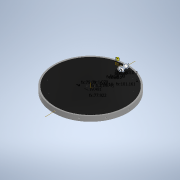
# Autodesk Inventor part: RotorBody
Saved by Autodesk Inventor 2022.2 (Build 262287000, 287)
## iProperties
Created: 2022-07-28
Part Number: RotorBody
Material: ABS Plastic
Document SubType Name: Modeling
Designer: ABL
Density: 1.06 g/cm^3
Appearance: Smooth - Black
Author: ABL
Autodesk Inventor part; units mm, degrees
ref_plane "YZ Plane" through (0, 0, 0) normal (1, 0, 0) x (0, 1, 0)
ref_plane "XZ Plane" through (0, 0, 0) normal (0, 1, 0) x (-1, 0, 0)
ref_plane "XY Plane" through (0, 0, 0) normal (0, 0, 1) x (1, 0, 0)
sketch "Sketch2" plane through (0, 0, 0) normal (0, 1, 0) x (-1, 0, 0)
  circle A0 centre (0, 0) radius 101.16113
  circle A1 centre (0, 0) radius 4.2
  dimension "d4" = 202.32226
  dimension "d101" = 8.4
  constraints: 2 centre point, 2 coincident
  measures "d4" diameter of A0
  measures "d101" diameter of A1
extrude "Extrusion1" add sketch "Sketch2" along normal blind 14.1
ref_plane "Work Plane4" through (-26.182427, 0, -97.714148) normal (-0.258819, 0, -0.9659258) x (0, -1, 0)
sketch "Sketch13" plane through (-27.256526, 0, -101.72274) normal (-0.258819, 0, -0.9659258) x (0, -1, 0)
  line L0 (-14.1, 101.16113) -> (-14.1, -101.16113) construction
  line L1 (0, 0) -> (-14.1, 0) construction
  line L2 (0, 0.05) -> (-14.1, 0.05)
  line L3 (-14.1, 0.05) -> (-14.1, -0.05)
  line L4 (-14.1, -0.05) -> (0, -0.05)
  line L5 (0, -0.05) -> (0, 0.05)
  line L6 (0, 0.05) -> (-14.1, -0.05) construction
  line L7 (-14.1, 0.05) -> (0, -0.05) construction
  point P0 (-7.05, 0)
  dimension "d136" = 0.1
  dimension "d139" = 7.05
  dimension "d140" = 2.05
  dimension "d141" = 4.2
  dimension "d142" = 3.8
  dimension "d146" = 4.1
  dimension "d147" = 4.3
  dimension "d153" = 4.2
  constraints: 8 end point, 2 parallel, 1 horizontal, 1 perpendicular
  measures "d153" distance of L2.end L3.end
sketch "Sketch10" plane through (0, 0, 0) normal (0, -1, 0) x (1, 0, 0)
  line L0 (0, 0) -> (-27.256526, -101.72274)
  line L1 (0, 0) -> (105.31113, 0) construction
  arc A0 (-27.256526, -101.72274) -> (30.042126, -100.935151) centre (0, 0) ccw
  line L2 (0, 0) -> (30.042126, -100.935151)
  line L3 (0, 0) -> (-27.256526, -101.72274) construction
  dimension "d96" = 105.31113
  dimension "d97" = 105
  dimension "d98" = 31.575
  constraints: 8 end point, 2 point on circle, 1 centre point, 1 coincident, 1 equal length, 1 horizontal
  measures "d96" distance of L0.start L0.end
  measures "d97" angle of L0 L1
  measures "d98" angle of L3 L2
sketch "Sketch8" plane through (0, 0, 0) normal (0, 1, 0) x (-1, 0, 0)
  circle A0 centre (0, 0) radius 105.31113
  circle A1 centre (0, 0) radius 101.21113
  dimension "d81" = 210.62226
  dimension "d82" = 202.42226
  constraints: 2 centre point, 2 coincident
  measures "d81" diameter of A0
  measures "d82" diameter of A1
extrude "Extrusion2" add sketch "Sketch8" along normal blind 14.1 separate body
sketch "Sketch1" plane through (0, 0, 0) normal (0, 1, 0) x (-1, 0, 0)
  circle A0 centre (0, 0) radius 38.96113 construction
  arc A1 (-26.182427, -97.714148) -> (26.182427, -97.714148) centre (0, 0) ccw
  line L0 (0, 0) -> (26.182427, -97.714148)
  line L1 (0, 0) -> (101.16113, 0) construction
  line L2 (0, 0) -> (-26.182427, -97.714148)
  line L3 (26.182427, -97.714148) -> (10.083882, -37.633562)
  line L4 (-26.182427, -97.714148) -> (-10.083882, -37.633562)
  line L5 (-9.168017, -38.203527) -> (0.974298, -39.286784)
  line L6 (0.974298, -39.286784) -> (-5.419042, -99.14633)
  line L7 (-5.419042, -99.14633) -> (-15.561357, -98.063073)
  line L8 (-15.561357, -98.063073) -> (-9.168017, -38.203527)
  line L9 (0, 0) -> (0, -101.16113) construction
  line L10 (9.075232, -38.016047) -> (2.9495, -38.972812)
  line L11 (2.9495, -38.972812) -> (12.239385, -98.4517)
  line L12 (12.239385, -98.4517) -> (18.365118, -97.494934)
  line L13 (18.365118, -97.494934) -> (9.075232, -38.016047)
  line L14 (-4.098764, -38.744933) -> (0, 0) construction
  circle A2 centre (-2.049382, -19.372466) radius 2.6
  circle A3 centre (0, 0) radius 101.16113 construction
  line L15 (5.352348, -87.575309) -> (0.955193, -87.733517)
  line L16 (0.955193, -87.733517) -> (1.012724, -89.332482)
  line L17 (1.012724, -89.332482) -> (5.409878, -89.174274)
  line L18 (5.409878, -89.174274) -> (5.352348, -87.575309)
  line L19 (0, 0) -> (3.153771, -87.654413) construction
  line L20 (0.955193, -87.733517) -> (-4.141944, -87.189113) construction
  line L21 (5.352348, -87.575309) -> (10.417072, -86.78426) construction
  line L22 (3.211301, -89.253378) -> (3.637384, -101.095715) construction
  line L23 (-4.098764, -38.744933) -> (-5.150777, -48.689442) construction
  line L24 (5.381113, -88.374792) -> (0.983959, -88.532999) construction
  point P0 (6.012366, -38.49443)
  point P1 (3.182536, -88.453895)
  dimension "d0" = 77.92226
  dimension "d1" = 101.16113
  dimension "d2" = 75
  dimension "d3" = 30
  dimension "d7" = 10.2
  dimension "d8" = 60.2
  dimension "d9" = 6.2
  dimension "d10" = 60.2
  dimension "d11" = 2
  dimension "d15" = 1.07874
  dimension "d16" = 1.07874
  dimension "d17" = 5.2
  dimension "d66" = 4.4
  dimension "d67" = 1.6
  dimension "d79" = 90
  dimension "d80" = 11.85
  dimension "d108" = 19.48057
  dimension "d122" = 10
  constraints: 50 end point, 7 midpoint, 7 perpendicular, 7 point on circle, 4 parallel, 4 point on line, 3 centre point, 3 coincident, 2 collinear, 2 equal length, 2 tangent, 1 horizontal
  measures "d0" diameter of A0
  measures "d1" radius of A1
  measures "d2" angle of L0 L1
  measures "d3" angle of L2 L0
  measures "d7" distance of L6.end L7.end
  measures "d8" distance of L5.end L6.end
  measures "d9" distance of L12.end L11.end
  measures "d10" distance of L11.end L10.end
  measures "d11" distance of L10.end L5.end
  measures "d15" distance of L5.start L4.end
  measures "d16" distance of L3.end L10.start
  measures "d17" diameter of A2
  measures "d66" distance of L15.start L15.end
  measures "d67" distance of L15.end L16.end
  measures "d79" angle of L19 L15
  measures "d80" distance of L22.start L22.end
  measures "d108" distance of A0.centre A2.centre
  measures "d122" distance of L14.start L23.end
extrude "driveMagnet_slot" cut sketch "Sketch1" along normal blind 10.1 contours L5 L6 L7 L8 bodies 1
extrude "halbachMagnet_slot" cut sketch "Sketch1" along normal blind 12.1 contours L13 L12 L11 L10 bodies 1
sketch "Sketch4" plane through (-12.239385, 0, -98.4517) normal (0.154317, 0, 0.9880214) x (0.9880214, 0, -0.154317)
  line L0 (0, 0) -> (0, 12.1) projected
  line L1 (0, 2) -> (-6.2, 2)
  line L2 (-6.2, 2) -> (-6.2, 12.2)
  line L3 (-6.2, 12.2) -> (0, 12.2)
  line L4 (0, 12.2) -> (0, 2)
  line L5 (0, 0) -> (-6.2, 0) projected
  point P0 (-3.1, 0)
  point P1 (0, 12.1)
  dimension "d31" = 6.2
  dimension "halbachMagnet_slotHeight" = 10.2
  dimension "d33" = 2
  constraints: 8 end point, 2 parallel, 1 horizontal, 1 perpendicular, 1 point on line
  measures "d31" distance of L2.end L3.end
  measures "halbachMagnet_slotHeight" distance of L1.end L2.end
  measures "d33" distance between parallel lines of L5 L1
extrude "halbachMagnet_opening" cut sketch "Sketch4" against normal through all bodies 1
extrude "halbachMagnet_roof" add sketch "Sketch1" along normal blind 2 contours L13 L12 L11 L10 bodies 1
extrude "halbachMagnet_slotTopSurfaceIndent" cut sketch "Sketch1" along normal blind 0.2 contours L13 L12 L11 L10 bodies 1
extrude "sensorMagnet_slot" cut sketch "Sketch1" along normal blind 2.766667 contours A2 bodies 1
extrude "rotorBandNut_slot" cut sketch "Sketch1" against normal blind 9.2 from surface at 14.1 contours L18 L17 L16 L15 bodies 1
hole "rotorBandNut_removalHole" at (-3.182536, 0, -88.453895) direction (0, 1, 0) diameter 1.4 depth 4.9 bodies 1
pattern_circular "Sketch1_Pattern" count 12 over 360 about axis through (0, -10, 0) along (0, 1, 0) of "rotorBandNut_removalHole", "rotorBandNut_slot", "sensorMagnet_slot", "halbachMagnet_roof", "halbachMagnet_opening", "halbachMagnet_slot", "driveMagnet_slot", "halbachMagnet_slotTopSurfaceIndent" bodies 1
sketch "Sketch7" plane through (-5.352348, 0, -87.575309) normal (-0.0359563, 0, -0.9993534) x (-0.9993534, 0, 0.0359563)
  line L0 (-2.2, 4.9) -> (-2.2, 7) construction
  line L1 (-4.4, 4.9) -> (0, 4.9) projected
  point P0 (-2.2, 0)
  dimension "d71" = 2.1
  constraints: 2 end point, 1 coincident, 1 midpoint, 1 vertical
  measures "d71" distance of L0.start L0.end
ref_plane "Work Plane2" through (-3.786602, 0, -105.243032) normal (0.0359563, 0, 0.9993534) x (0, 1, 0)
ref_plane "Work Plane1" through (-5.352348, 9.5, -87.575309) normal (0.0359563, 0, 0.9993534) x (0, 1, 0)
sketch "Sketch9" plane through (-3.786602, 0, -105.243032) normal (0.0359563, 0, 0.9993534) x (0, 1, 0)
  line L0 (0, 0) -> (7.05, 0) construction
  dimension "d85" = 7.05
  constraints: 2 coincident, 2 end point, 1 horizontal
  measures "d85" distance of L0.start L0.end
hole "rotorBandBolt_hole" at (-3.786602, 7.05, -105.243032) direction (0.0359563, 0, 0.9993534) diameter 2.4 depth 24 counterbore diameter 4.08 counterbore depth 2.1 bodies 2 1
sketch "Sketch18" plane through (-0.955193, 4.9, -87.733517) normal (-0.0359563, 0, -0.9993534) x (-0.9993534, 0, 0.0359563)
  line L0 (0, 0.879829) -> (0, 3.420171)
  line L1 (0, 3.420171) -> (2.2, 4.690341)
  line L2 (2.2, 4.690341) -> (4.4, 3.420171)
  line L3 (4.4, 3.420171) -> (4.4, 0.879829)
  line L4 (4.4, 0.879829) -> (2.2, -0.390341)
  line L5 (2.2, -0.390341) -> (0, 0.879829)
  circle A0 centre (2.2, 2.15) radius 1.2
  line L6 (0, 9.2) -> (4.4, 9.2)
  line L7 (0, 9.2) -> (0, 0)
  line L8 (0, 0) -> (4.4, 0)
  line L9 (4.4, 0) -> (4.4, 9.2)
  point P0 (2.2, -4.9)
  dimension "d176" = 4.4
  constraints: 12 end point, 1 coincident, 1 vertical, 13 other
  measures "d176" distance between parallel lines of L3 L0
extrude "rotorBandNut_hexCutaway" cut sketch "Sketch18" along normal up to surface (1.6 mm away) contours L0 L1 L2 L3 L4 L8 L5 | L8 L4 L5 | A0 bodies 1
pattern_circular "BoltHoles" count 12 over 360 about axis through (0, -10, 0) along (0, 1, 0) of "rotorBandBolt_hole", "rotorBandNut_hexCutaway" bodies 1 2
sketch "Sketch11" plane through (0, 0, 0) normal (0, -1, 0) x (1, 0, 0)
  circle A0 centre (0, 0) radius 9
  circle A1 centre (0, 0) radius 8
  dimension "d102" = 18
  dimension "d105" = 16
  constraints: 2 centre point, 2 coincident
  measures "d102" diameter of A0
  measures "d105" diameter of A1
extrude "flangeBearing_flangeInset" cut sketch "Sketch11" against normal blind 1.4 bodies 1
extrude "flangeBearing_bodyInset" cut sketch "Sketch11" against normal blind 5.2 contours A1 bodies 1
ref_plane "Work Plane3" through (0, 7.05, 0) normal (0, -1, 0) x (1, 0, 0)
mirror "flangeBearing_mirror" about plane through (0, 7.05, 0) normal (0, -1, 0) of "flangeBearing_flangeInset", "flangeBearing_bodyInset" bodies 1
hole "halbachMagnet_removalHole" at (-6.012366, 0, -38.49443) direction (0, 1, 0) diameter 2 depth 12.1 bodies 1
sketch "Sketch12" plane through (-9.075232, 2, -38.016047) normal (-0.154317, 0, -0.9880214) x (-0.9880214, 0, 0.154317)
  line L0 (-6.2, 0) -> (0, 0) projected
  line L1 (-3.1, 0) -> (-3.1, -2) construction
  line L2 (-3.1, -2) -> (-4.1, -2)
  line L3 (-4.1, -2) -> (-4.1, 0)
  line L4 (-4.1, 0) -> (-3.1, 0)
  line L5 (-3.1, -2) -> (-2.1, -2)
  line L6 (-2.1, -2) -> (-2.1, 0)
  line L7 (-2.1, 0) -> (-3.1, 0)
  point P0 (-2.1, 0)
  point P1 (-4.1, 0)
  dimension "d116" = 1
  constraints: 14 end point, 2 parallel, 2 symmetric about line, 1 midpoint, 1 perpendicular, 1 vertical
  measures "d116" distance of L1.end L2.end
extrude "halbachMagnet_removalChannel" cut sketch "Sketch12" along normal blind 10 bodies 1
hole "driveMagnet_removalHole" at (5.150777, 0, -48.689442) direction (0, 1, 0) diameter 2 depth 14.1 bodies 1
pattern_circular "Circular Pattern3" count 12 over 360 about axis through (0, -10, 0) along (0, 1, 0) of "halbachMagnet_removalHole", "halbachMagnet_removalChannel", "driveMagnet_removalHole" bodies 1
sketch "Sketch17" plane through (0, 0, 0) normal (0, -1, 0) x (1, 0, 0)
  circle A0 centre (0, 0) radius 8 construction
  line L0 (0, 0) -> (27.256526, -101.72274) construction
  circle A1 centre (0, 0) radius 105.31113 construction
  line L1 (0, 0) -> (105.31113, 0) construction
  arc A2 (27.256526, -101.72274) -> (101.72274, -27.256526) centre (0, 0) ccw
  line L2 (0, 0) -> (101.72274, -27.256526)
  line L3 (0, 0) -> (27.256526, -101.72274) construction
  arc A3 (-74.466214, -74.466214) -> (27.256526, -101.72274) centre (0, 0) ccw
  line L4 (0, 0) -> (-74.466214, -74.466214)
  line L5 (0, 0) -> (27.256526, -101.72274) construction
  dimension "d154" = 75
  dimension "d155" = 60
  dimension "d156" = 60
  constraints: 12 end point, 7 point on circle, 2 centre point, 2 coincident, 2 concentric, 1 equal length, 1 horizontal
  measures "d154" angle of L0 L1
  measures "d155" angle of L3 L2
  measures "d156" angle of L4 L5
extrude "rotorBand_printingExport" [suppressed]
equation "\"d4\" = 2 * rotorRadius"
equation "\"d5\" = rotorThickness"
equation "\"d0\" = 2 * driveMagnet_centerSpacingRadius"
equation "\"d1\" = rotorRadius"
equation "\"d7\" = driveMagnet_width + 2 * gap"
equation "\"d8\" = driveMagnet_length + 2 * gap"
equation "\"d10\" = halbachMagnet_length + 2 * gap"
equation "\"d11\" = wallgap"
equation "\"d16\" = d15"
equation "\"d17\" = sensorMagnet_diameter + 2 * gap"
equation "\"d20\" = gap + halbachMagnet_width + wallgap"
equation "\"d33\" = wallgap"
equation "\"d36\" = wallgap"
equation "\"d22\" = sensorMagnet_height + gap"
equation "\"d68\" = 0.5 * rotorBandSquareNut_sideLength + 0.5 * halbachMagnet_slotHeight + wallgap + gap"
equation "\"d71\" = 0.5 * rotorBandSquareNut_sideLength + gap"
equation "\"gap\" = 0.1"
equation "\"airgap\" = 0.4"
equation "\"driveMagnet_height\" = 5"
equation "\"halbachMagnet_width\" = 10"
equation "\"halbachMagnet_height\" = 3"
equation "\"sensorMagnet_diameter\" = 5"
equation "\"sensorMagnet_height\" = 2.66667"
equation "\"wallgap\" = 2"
equation "\"driveMagnet_centerSpacingRadius\" = 38.96113"
equation "\"rotorThickness\" = 14.1"
equation "\"shaftDiameter\" = 8"
equation "\"flangeBearing_outerDiameter\" = 16"
equation "\"flangeBearing_innerDiameter\" = shaftDiameter"
equation "\"flangeBearing_height\" = 5"
equation "\"flangeBearing_flangeHeight\" = 1"
equation "\"flangeBearing_flangeDiameter\" = 18"
equation "\"statorThickness\" = 16"
equation "\"rotor_mountingLipHeight\" = 8"
equation "\"rotorRadius\" = 101.16113"
equation "\"rotorBandSquareNut_sideLength\" = 4"
equation "\"rotorBandHexNut_height\" = 1.2"
equation "\"rotorBandHexNut_sideToSide\" = 4"
equation "\"rotorBandSquareNut_height\" = 1.2"
equation "\"rotorBandBolt_headHeight\" = 2"
equation "\"rotorBandBolt_headDiameter\" = 3.98"
equation "\"rotorBandBolt_diameter\" = 2"
equation "\"rotorBandThickness\" = 4.1"
equation "\"flangeCoupling_collarOuterDiameter\" = 16"
equation "\"flangeCoupling_flangeHoleEdgeToEdge\" = 2.05"
equation "\"flangeCoupling_innerDiameter\" = 8"
equation "\"flangeCoupling_flangeHoleDiameter\" = 3.9"
equation "\"flangeCoupling_flangeHeight\" = 3.1"
equation "\"flangeCoupling_flangeDiameter\" = 32"
equation "\"flangeCoupling_height\" = 13.1"
equation "\"flangeCoupling_mountHoleDiameter\" = 3.9"
equation "\"flangeCoupling_mountHoleEdgeToEdge\" = 2.05"
equation "\"statorRadius\" = 99.16113"
equation "\"coilThickness\" = 12"
equation "\"statorMountBolt_diameter\" = 4"
equation "\"statorMountBolt_headDiameter\" = 7"
equation "\"statorMountBolt_headHeight\" = 4"
equation "\"statorMountBolt_shaftLength\" = 17.1"
equation "\"statorMountHexNut_height\" = 4"
equation "\"statorMountHexNut_sideToSide\" = 8"
equation "\"sensorMagnet_ringRadius\" = 23.48057"
equation "\"coil_percentCoverage\" = 0.6"
equation "\"statorSpokeDegrees\" = 4deg"
equation "\"coil_bulge\" = 3"
equation "\"statorCoilBolt_shaftLength\" = 12"
equation "\"statorCoilHexNut_height\" = 1.2"
equation "\"statorCoilBolt_headHeight\" = 2"
equation "\"statorCoilBolt_diameter\" = 2"
equation "\"statorCoilBolt_headDiameter\" = 3.98"
equation "\"statorCoilHexNut_sideToSide\" = 4"
equation "\"magnetWire_outerDiameter\" = 0.8128"
equation "\"printingLayerHeight\" = 0.2"
equation "\"circuitBoard_height\" = 1.6"
equation "\"hallEffectSensor_width\" = 1.6"
equation "\"hallEffectSensor_length\" = 3"
equation "\"hallEffectSensor_height\" = 1.1"
equation "\"hallEffectSensor_pinLength\" = 0.6"
equation "\"circuitboardMountHexNut_height\" = 1.2"
equation "\"circuitboardMountHexNut_sideToSide\" = 4"
equation "\"circuitboardMountBolt_headHeight\" = 2"
equation "\"circuitboardMountBolt_shaftLength\" = 12"
equation "\"circuitboardMountBolt_diameter\" = 2"
equation "\"circuitboardMountBolt_headDiameter\" = 3.98"
equation "\"statorShellBolt_headDiameter\" = 5.68"
equation "\"statorShellHexNut_height\" = 2.3"
equation "\"statorShellBolt_shaftLength\" = 12.6"
equation "\"statorShellBolt_headHeight\" = 3"
equation "\"statorShellHexNut_sideToSide\" = 5.3"
equation "\"statorShellBolt_diameter\" = 3"
equation "\"statorShellBolt_countersinkDepth\" = 3.4"
equation "\"driveMagnet_width\" = 10"
equation "\"driveMagnet_length\" = 60"
equation "\"halbachMagnet_length\" = 60"
